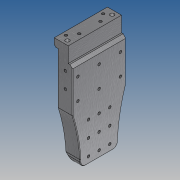
# Autodesk Inventor part: J008083
Saved by Autodesk Inventor 2018.3 (Build 223284000, 284)
## iProperties
Created: 2014-12-15
Material: ALUMINUM, 6061-T651
Vendor: HHMI: JFRC - ID&F
Document SubType Name: Modeling
Designer: ARNOLDJ
Density: 2.7 g/cm^3
Mass: 360.292 g
Surface Area: 312.552 cm^2
Volume: 133.442 cm^3
Description: MBS OUTER POSARM NO GONIO
Appearance: Polished Brushed
Project: COMMON
Part Number: J008083
RuleStatus: InUse
AfterDocSave0: file://Part Number Cleaner
LAB/DEPT: PACHITARIU (LAB)
REQUESTING SCIENTIST: PACHITARIU, MARIUS
SURFACE ROUGHNESS: 63 Ra
DESIGN DEPARTMENT: HHMI: JRC - ID&F
SPECIAL FINISH: ANODIZE PER MIL-A-8625F, TYPE II, CLASS 2 (BLACK)
ALTERED ITEM PART NUMBER: N/A
ALTERED ITEM VENDOR: N/A
ALTERED ITEM DESCRIPTION: N/A
Revision Number: -
Autodesk Inventor part; units mm, degrees
ref_plane "XZ Plane" through (0, 0, 0) normal (0, 1, 0) x (-1, 0, 0)
sketch "Sketch1" plane through (0, 0, 0) normal (0, 0, 1) x (1, 0, 0)
  line L0 (0, 105.3389) -> (0, -75.1637) projected
  line L1 (-19.05, 0) -> (3.175, 0) projected
  line L2 (-15.875, -49.3776) -> (-15.875, 79.5528)
  line L3 (0, -49.3776) -> (0, 79.5528)
  line L4 (-15.875, 79.5528) -> (0, 79.5528)
  line L5 (0, -49.3776) -> (-15.875, -49.3776)
  line L6 (-7.9375, 79.5528) -> (-7.9375, -49.3776) construction
  point P0 (0, 0)
  dimension "d5" = 15.875
  dimension "d67" = 0
  dimension "d118" = 49.3776
  dimension "d119" = 79.5528
  constraints: 10 end point, 2 horizontal, 2 midpoint, 1 perpendicular, 1 vertical
  measures "d5" distance between parallel lines of L2 L3
  measures "d67" distance between parallel lines of L0 L3
  measures "d118" distance between parallel lines of L5 L1
  measures "d119" distance between parallel lines of L1 L4
extrude "Extrusion1" add sketch "Sketch1" along normal mid plane 63.5
sketch "Sketch25" plane through (0, 0, 0) normal (0, 0, 1) x (1, 0, 0)
  line L0 (-15.875, 79.5528) -> (0, 79.5528) projected
  line L1 (0, 79.5528) -> (0, -49.3776) projected
  line L2 (0, 79.5528) -> (-5.08, 79.5528)
  line L3 (-5.08, 79.5528) -> (-5.08, 61.3156)
  line L4 (-5.08, 61.3156) -> (0, 61.3156)
  line L5 (0, 61.3156) -> (0, 79.5528)
  point P0 (0, 0)
  dimension "d280" = 5.08
  dimension "d281" = 18.2372
  constraints: 8 end point, 2 parallel, 1 horizontal, 1 perpendicular
  measures "d280" distance of L3.end L4.end
  measures "d281" distance of L2.end L3.end
extrude "Extrusion13" cut sketch "Sketch25" along normal mid plane 76.2
sketch "Sketch26" plane through (0, 0, 0) normal (0, 0, 1) x (1, 0, 0)
  line L0 (-15.875, 79.5528) -> (0, 79.5528) projected
  line L1 (-15.875, -49.3776) -> (-15.875, 79.5528) projected
  line L2 (-15.875, 79.5528) -> (-21.844, 79.5528)
  line L3 (-21.844, 79.5528) -> (-21.844, 70.6628)
  line L4 (-21.844, 70.6628) -> (-15.875, 70.6628)
  line L5 (-15.875, 70.6628) -> (-15.875, 79.5528)
  line L6 (-15.875, 70.6628) -> (-17.145, 70.6628)
  line L7 (-17.145, 70.6628) -> (-17.145, -49.3776)
  line L8 (-17.145, -49.3776) -> (-15.875, -49.3776)
  line L9 (-15.875, -49.3776) -> (-15.875, 70.6628)
  line L10 (0, -49.3776) -> (-15.875, -49.3776) projected
  point P0 (0, 0)
  point P1 (-5.08, 79.5528)
  point P2 (-15.875, 56.6928)
  dimension "d284" = 5.969
  dimension "d285" = 8.89
  dimension "d313" = 22.86
  dimension "d318" = 1.27
  dimension "d415" = 0
  constraints: 16 end point, 4 parallel, 2 horizontal, 2 perpendicular, 1 point on line
  measures "d284" distance of L3.end L4.end
  measures "d285" distance of L2.end L3.end
  measures "d313" distance from line of L0 point (-15.875, 56.693)
  measures "d318" distance of L7.end L8.end
  measures "d415" distance from line of L7.end L10
extrude "Extrusion14" add sketch "Sketch26" along normal up to surface (63.5 mm away) from surface at -31.75
sketch "Sketch20" plane through (0, 0, 0) normal (1, 0, 0) x (0, 1, 0)
  line L0 (-49.3776, -31.75) -> (-49.3776, 31.75) projected
  line L1 (-49.3776, -31.75) -> (79.5528, -31.75) projected
  line L2 (-41.7576, 12.7) -> (-3.6576, 12.7) construction
  line L3 (-3.6576, 12.7) -> (-3.6576, -12.7) construction
  line L4 (-3.6576, -12.7) -> (-41.7576, -12.7) construction
  line L5 (-41.7576, -12.7) -> (-41.7576, 12.7) construction
  line L6 (-76.6877, 0) -> (105.5929, 0) construction
  line L7 (21.7424, 25.4) -> (21.7424, -25.4)
  line L8 (21.7424, 25.4) -> (47.1424, 25.4)
  line L9 (47.1424, 25.4) -> (47.1424, -25.4)
  line L10 (47.1424, -25.4) -> (21.7424, -25.4)
  line L11 (21.7424, -25.4) -> (21.7424, 25.4)
  line L12 (26.88, 21.59) -> (43.3324, 21.59)
  line L13 (43.3324, 21.59) -> (43.3324, 3.81)
  line L14 (43.3324, 3.81) -> (26.88, 3.81)
  line L15 (26.88, 3.81) -> (26.88, 21.59)
  line L16 (25.5524, -3.81) -> (43.3324, -3.81)
  line L17 (43.3324, -3.81) -> (43.3324, -21.59)
  line L18 (43.3324, -21.59) -> (25.5524, -21.59)
  line L19 (25.5524, -21.59) -> (25.5524, -3.81)
  line L20 (0, 44.45) -> (0, -44.45) projected
  point P0 (0, 0)
  point P1 (21.7424, 0)
  point P2 (47.1424, 0)
  point P3 (-22.7076, 12.7)
  point P4 (-22.7076, -12.7)
  point P5 (-22.7076, 0)
  point P6 (-41.7576, 0)
  point P7 (-3.6576, 0)
  dimension "d350" = 25.4
  dimension "d351" = 38.1
  dimension "d352" = 12.7
  dimension "d354" = 25.4
  dimension "d355" = 50.8
  dimension "d356" = 25.4
  dimension "d360" = 3.81
  dimension "d361" = 3.81
  dimension "d362" = 3.81
  dimension "d363" = 3.81
  dimension "d364" = 7.62
  dimension "d365" = 3.81
  dimension "d366" = 16.4523
  dimension "d418" = 41.7576
  constraints: 34 end point, 8 coincident, 8 parallel, 6 midpoint, 4 horizontal, 4 perpendicular, 4 point on line, 1 symmetric about line, 1 vertical, 1 other
  measures "d350" distance of L4.end L2.start
  measures "d351" distance of L2.start L2.end
  measures "d352" distance between parallel lines of L6 L2
  measures "d354" distance between parallel lines of L7 L3
  measures "d355" distance of L7.start L7.end
  measures "d356" distance of L8.start L8.end
  measures "d360" distance between parallel lines of L11 L19
  measures "d361" distance between parallel lines of L9 L13
  measures "d362" distance between parallel lines of L8 L12
  measures "d363" distance between parallel lines of L10 L18
  measures "d364" distance between parallel lines of L14 L16
  measures "d365" distance between parallel lines of L14 L6
  measures "d366" distance of L12.start L12.end
  measures "d418" distance from line of L20 point (-41.758, 12.7)
hole "Hole10" at (0, -41.7576, 12.7) at (0, -41.7576, -12.7) at (0, -3.6576, 12.7) at (0, -3.6576, -12.7) at (0, 21.7424, -25.4) at (0, 47.1424, -25.4) at (0, 47.1424, 25.4) at (0, 21.7424, 25.4) at (0, 47.1424, 0) at (0, 21.7424, 0) at (0, -41.7576, 0) at (0, -22.7076, -12.7) at (0, -22.7076, 0) at (0, -22.7076, 12.7) at (0, -3.6576, 0) direction (-1, 0, 0) diameter 3.2512 depth 12.7 tip angle 118
ref_plane "Work Plane3" through (-56.8706, -53.1876, 22.5) normal (0, -1, 0) x (1, 0, 0)
ref_plane "Work Plane2" through (-38.862, 0, 0) normal (1, 0, 0) x (0, 1, 0)
sketch "Sketch23" plane through (-15.875, 79.5528, 31.75) normal (0, 1, 0) x (1, 0, 0)
  line L0 (4.7625, 0) -> (4.7625, 63.5) construction
  line L1 (15.875, 63.5) -> (15.875, 0) projected
  point P0 (15.875, 31.75)
  point P1 (4.7625, 5.08)
  point P2 (4.7625, 19.05)
  point P3 (4.7625, 44.45)
  point P4 (4.7625, 58.42)
  point P5 (-1.5875, 9.525)
  point P6 (-1.5875, 53.975)
  dimension "d260" = 12.7
  dimension "d261" = 25.4
  dimension "d262" = 26.67
  dimension "d263" = 53.34
  dimension "d289" = 44.45
  dimension "d290" = 22.225
  dimension "d291" = 6.35
  dimension "d319" = 11.1125
  constraints: 4 point on line, 2 end point, 1 vertical alignment
  measures "d260" vertical distance of point (15.875, 31.75) point (4.763, 19.05)
  measures "d261" distance of point (4.763, 44.45) point (4.763, 19.05)
  measures "d262" vertical distance of point (15.875, 31.75) point (4.763, 5.08)
  measures "d263" distance of point (4.763, 5.08) point (4.763, 58.42)
  measures "d289" distance of point (-1.587, 53.975) point (-1.587, 9.525)
  measures "d290" vertical distance of point (15.875, 31.75) point (-1.587, 9.525)
  measures "d291" distance from line of point (-1.587, 9.525) L0
  measures "d319" distance between parallel lines of L0 L1
hole "Hole12" at (-11.1125, 79.5528, 26.67) at (-11.1125, 79.5528, -26.67) direction (0, -1, 0) diameter 4.7498 depth 22.86 tip angle 118 counterbore diameter 4.7879 counterbore depth 5.08
hole "Hole13" at (-17.4625, 79.5528, 22.225) at (-17.4625, 79.5528, -22.225) at (-11.1125, 79.5528, 12.7) at (-11.1125, 79.5528, -12.7) direction (0, -1, 0) diameter 3.2512 depth 14.605 tip angle 118
sketch "Sketch37" plane through (0, -49.3776, 31.75) normal (1, 0, 0) x (0, 0, -1)
  point P0 (31.75, 49.3776)
sketch "Sketch24" plane through (0, 0, 0) normal (1, 0, 0) x (0, 1, 0)
  line L0 (-53.1876, -22.5) -> (-40.4876, -22.5)
  line L1 (9.6224, -31.75) -> (-53.1876, -31.75)
  line L2 (-53.1876, -31.75) -> (-53.1876, -22.5)
  line L3 (-40.4876, -22.5) -> (-40.4876, -31.75) construction
  line L4 (19.8628, -31.75) -> (-53.1876, -31.75) construction
  line L5 (0, 83.1744) -> (0, -276.7964) projected
  line L6 (-191.8934, 0) -> (149.0556, 0) projected
  line L7 (100.3486, 0) -> (-143.1864, 0) construction
  arc A0 (9.6224, -31.75) -> (-40.4876, -22.5) centre (-52.0278, -225.372) ccw
  point P0 (0, 0)
  point P1 (-49.3776, -31.75)
  point P2 (19.8628, 31.75)
  dimension "d375" = 62.81
  dimension "d382" = 203.2
  dimension "d383" = 9.25
  dimension "d414" = 52.0278
  dimension "d419" = 40.4876
  constraints: 10 end point, 3 point on line, 2 point on circle, 1 centre point, 1 horizontal, 1 horizontal alignment, 1 parallel, 1 perpendicular
  measures "d375" distance of L1.start L1.end
  measures "d382" radius of A0
  measures "d383" distance of L1.end L0.start
  measures "d414" distance from line of L5 A0.centre
  measures "d419" distance from line of L5 L0.end
extrude "Extrusion12" cut sketch "Sketch24" against normal through all
mirror "Mirror1" about plane through (0, 0, 0) normal (0, 0, 1) of "Extrusion12"
chamfer "Chamfer6" distance 1.905 angle 45 1 edges at (-21.844, 70.6628, 0)
chamfer "Chamfer12" distance 8.89 angle 45 1 edges at (-17.145, -49.3776, 0)
fillet "Fillet17" radius 6.35 2 edges at (-4.1275, -49.3776, 22.5) (-4.1275, -49.3776, -22.5)
chamfer "Chamfer11" distance 0.635 angle 45 9 edges at (0, -41.7576, -22.5) (0, -47.5177, -20.6401) (0, -49.3776, 0) (0, -47.5177, 20.6401) (0, -41.7576, 22.5) (0, 35.469, -31.75) (0, 35.469, 31.75) (0, -15.1415, -25.548) (0, -15.1415, 25.548)
sketch "Sketch39" plane through (0, 0, -31.75) normal (0, 0, -1) x (-1, 0, 0)
  line L0 (17.145, -49.3776) -> (17.145, 70.6628) projected
  line L1 (8.5725, 51.9684) -> (8.5725, 32.9184) construction
  line L2 (0, 61.3156) -> (0, 9.721) construction
  circle A0 centre (8.5725, 32.9184) radius 2.0003 construction
  circle A1 centre (8.5725, 51.9684) radius 2.0003 construction
  line L3 (0.635, 9.6224) -> (0.635, 61.3156) construction
  line L4 (0.635, 9.6224) -> (17.145, 9.6224) construction
  line L5 (17.145, 9.6224) -> (17.145, 70.6628) construction
  line L6 (17.145, 70.6628) -> (19.939, 70.6628) construction
  line L7 (21.844, 72.5678) -> (19.939, 70.6628) construction
  line L8 (21.844, 72.5678) -> (21.844, 79.5528) construction
  line L9 (21.844, 79.5528) -> (5.08, 79.5528) construction
  line L10 (5.08, 79.5528) -> (5.08, 61.3156) construction
  line L11 (5.08, 61.3156) -> (0.635, 61.3156) construction
  line L12 (-4.3688, 0) -> (26.2128, 0) projected
  point P0 (0, 0)
  point P1 (0, 58.1406)
  dimension "d391" = 8.5725
  dimension "d392" = 17.145
  dimension "d394" = 4.0005
  dimension "d395" = 4.0005
  dimension "d404" = 19.05
  dimension "d405" = 27.5844
  dimension "d417" = 32.9184
  constraints: 4 coincident, 2 centre point, 2 end point, 1 vertical
  measures "d391" distance between parallel lines of L1 L0
  measures "d392" distance between parallel lines of L2 L0
  measures "d394" diameter of A0
  measures "d395" diameter of A1
  measures "d404" distance of L1.start L1.end
  measures "d405" distance from line of L9 point (8.572, 51.968)
  measures "d417" distance from line of L1.end L12
hole "Hole14" at (-8.5725, 32.9184, -31.75) at (-8.5725, 51.9684, -31.75) direction (0, 0, 1) diameter 3.2512 depth 12.7 tip angle 118
sketch "Sketch40" plane through (0, 0, 31.75) normal (0, 0, 1) x (1, 0, 0)
  circle A0 centre (-8.5725, 51.9684) radius 1.6256 projected
  circle A1 centre (-8.5725, 32.9184) radius 1.6256 projected
  point P0 (0, 0)
  constraints: 2 coincident
hole "Hole15" at (-8.5725, 51.9684, 31.75) at (-8.5725, 32.9184, 31.75) direction (0, 0, -1) diameter 3.2512 depth 12.7 tip angle 118
chamfer "Chamfer13" distance 3.175 angle 45 1 edges at (0, 61.3156, 0)
body "Solid1"
